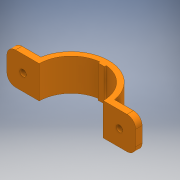
# Autodesk Inventor part: Motor Mount C-Clamp Top
Saved by Autodesk Inventor 2018 (Build 220112000, 112)
## iProperties
Created: 2018-01-11
Part Number: Motor Mount C-Clamp Top
Material: Generic
Document SubType Name: Modeling
Designer: Moochster
Density: 1 g/cm^3
Appearance: Orange
Author: Moochster
Autodesk Inventor part; units mm, degrees
ref_plane "YZ Plane" through (0, 0, 0) normal (1, 0, 0) x (0, 1, 0)
ref_plane "XZ Plane" through (0, 0, 0) normal (0, 1, 0) x (-1, 0, 0)
ref_plane "XY Plane" through (0, 0, 0) normal (0, 0, 1) x (1, 0, 0)
sketch "Sketch1" plane through (0, 0, 0) normal (0, 0, 1) x (1, 0, 0)
  arc A0 (14.865, 0) -> (-14.865, 0) centre (0, 0) ccw
  arc A1 (17.1039, 3) -> (-17.1039, 3) centre (0, 0) ccw
  line L0 (-17.1039, 3) -> (-29.865, 3)
  line L1 (-29.865, 3) -> (-29.865, 0)
  line L2 (-29.865, 0) -> (-14.865, 0)
  line L3 (14.865, 0) -> (29.865, 0)
  line L4 (29.865, 0) -> (29.865, 3)
  line L5 (29.865, 3) -> (17.1039, 3)
  arc A2 (1.4092, 13.8937) -> (-1.4092, 13.8937) centre (0, 0) ccw
  line L6 (-1.4092, 13.8937) -> (-1.5, 14.7891)
  line L7 (1.4092, 13.8937) -> (1.5, 14.7891)
  point P0 (0, 13.965)
  dimension "d0" = 3
  dimension "d1" = 14.865
  dimension "d3" = 2.5
  dimension "d8" = 15
  dimension "d17" = 0.9
  dimension "d18" = 3
  constraints: 16 end point, 9 point on circle, 4 horizontal, 3 centre point, 3 horizontal alignment, 2 concentric, 2 equal length, 2 line through centre, 2 perpendicular, 1 coincident, 1 vertical alignment
  measures "d0" distance of L3.end L4.end
  measures "d1" radius of A0
  measures "d3" radial gap between concentric circles of A0 A1
  measures "d8" distance of L3.start L3.end
  measures "d17" radial gap between concentric circles of A0 A2
  measures "d18" distance of L7.end L6.end
extrude "Extrusion1" add sketch "Sketch1" along normal blind 15
sketch "Sketch2" plane through (-29.865, 0, 0) normal (0, -1, 0) x (1, 0, 0)
  line L0 (0, 15) -> (15, 15) projected
  line L1 (0, 0) -> (0, 15) projected
  point P0 (29.865, 0)
  point P1 (7.5, 7.5)
  point P2 (7.5, 15)
  point P3 (0, 7.5)
  constraints: 2 midpoint, 1 horizontal alignment, 1 vertical alignment
hole "Hole1" at (-22.365, 0, 7.5) direction (0, 1, 0) diameter 3 end through all
mirror "Mirror1" about plane through (0, 0, 0) normal (1, 0, 0) of "Hole1"
fillet "Fillet1" radius 4 4 edges at (-29.865, 1.5, 0) (-29.865, 1.5, 15) (29.865, 1.5, 15) (29.865, 1.5, 0)
body "Solid1"
